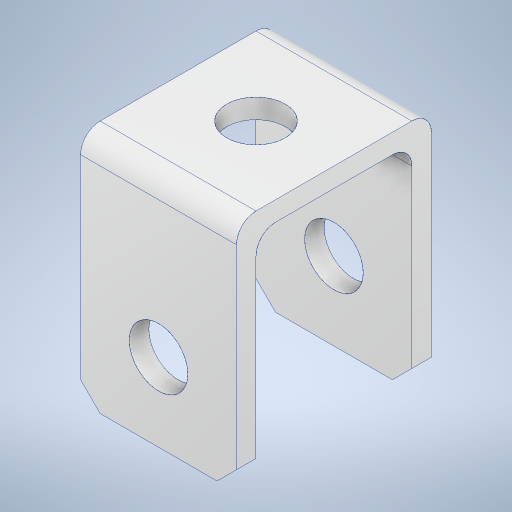
# Autodesk Inventor part: pnuematic bracket
Saved by Autodesk Inventor 2023 (Build 270158000, 158)
## iProperties
Created: 2022-07-24
Part Number: pnuematic bracket
Material: Aluminum 6061
Document SubType Name: Modeling
Designer: aaron
Density: 2.7 g/cm^3
Appearance: Aluminum - Flat
Author: aaron
Autodesk Inventor part; units mm, degrees
ref_plane "YZ Plane" through (0, 0, 0) normal (1, 0, 0) x (0, 1, 0)
ref_plane "XZ Plane" through (0, 0, 0) normal (0, 1, 0) x (-1, 0, 0)
ref_plane "XY Plane" through (0, 0, 0) normal (0, 0, 1) x (1, 0, 0)
sketch "Sketch1" plane through (0, 0, 0) normal (0, 1, 0) x (-1, 0, 0)
  line L0 (-6.35, -6.35) -> (6.35, -6.35)
  line L1 (6.35, -6.35) -> (6.35, 6.35)
  line L2 (6.35, 6.35) -> (-6.35, 6.35)
  line L3 (-6.35, 6.35) -> (-6.35, -6.35)
  line L4 (-6.35, -6.35) -> (6.35, 6.35) construction
  line L5 (6.35, -6.35) -> (-6.35, 6.35) construction
  point P0 (0, 0)
  dimension "d0" = 12.7
  dimension "d1" = 12.7
  constraints: 12 end point, 2 midpoint, 2 parallel, 1 horizontal, 1 perpendicular
  measures "d0" distance of L2.end L1.end
  measures "d1" distance of L1.end L0.end
extrude "Extrusion1" add sketch "Sketch1" along normal blind 1.5875
sketch "Sketch2" plane through (0, 1.5875, 0) normal (0, 1, 0) x (1, 0, 0)
  circle A0 centre (0, 0) radius 2.3812
  dimension "d4" = 4.7625
  constraints: 1 centre point, 1 coincident
  measures "d4" diameter of A0
extrude "Extrusion2" cut sketch "Sketch2" against normal blind 1.5875
sketch "Sketch3" plane through (0, 1.5875, 0) normal (0, 1, 0) x (1, 0, 0)
  line L0 (-6.35, -6.35) -> (6.35, -6.35) projected
  line L1 (-6.35, -6.35) -> (6.35, -6.35)
  line L2 (6.35, -6.35) -> (6.35, -7.9375)
  line L3 (6.35, -7.9375) -> (-6.35, -7.9375)
  line L4 (-6.35, -7.9375) -> (-6.35, -6.35)
  line L5 (6.35, -6.35) -> (6.35, 6.35) projected
  line L6 (6.35, 6.35) -> (-6.35, 6.35)
  line L7 (-6.35, 6.35) -> (-6.35, 7.9375)
  line L8 (-6.35, 7.9375) -> (6.35, 7.9375)
  line L9 (6.35, 7.9375) -> (6.35, 6.35)
  point P0 (0, 0)
  dimension "d7" = 12.7
  dimension "d8" = 1.5875
  dimension "d9" = 12.7
  dimension "d10" = 1.5875
  constraints: 16 end point, 4 parallel, 2 horizontal, 2 perpendicular
  measures "d7" distance of L2.end L3.end
  measures "d8" distance of L1.end L2.end
  measures "d9" distance of L7.end L8.end
  measures "d10" distance of L6.end L7.end
extrude "Extrusion3" add sketch "Sketch3" against normal blind 19.05
sketch "Sketch4" plane through (-6.35, 1.5875, 7.9375) normal (0, 0, 1) x (1, 0, 0)
  circle A0 centre (6.35, -12.7) radius 2.3813
  line L0 (12.7, 0) -> (12.7, -19.05) projected
  line L1 (12.7, -19.05) -> (0, -19.05) projected
  point P0 (6.35, -1.5875)
  dimension "d13" = 4.7625
  dimension "d14" = 6.35
  dimension "d15" = 6.35
  constraints: 1 centre point
  measures "d13" diameter of A0
  measures "d14" distance from line of L0 A0.centre
  measures "d15" distance from line of L1 A0.centre
extrude "Extrusion4" cut sketch "Sketch4" against normal blind 19.05
fillet "Fillet1" radius 1.5875 4 edges at (0, 1.5875, 7.9375) (0, 0, 6.35) (0, 0, -6.35) (0, 1.5875, -7.9375)
chamfer "Chamfer1" distance 1.5875 angle 45 4 edges at (6.35, -17.4625, 7.1437) (6.35, -17.4625, -7.1437) (-6.35, -17.4625, -7.1437) (-6.35, -17.4625, 7.1437)
body "Solid1"
